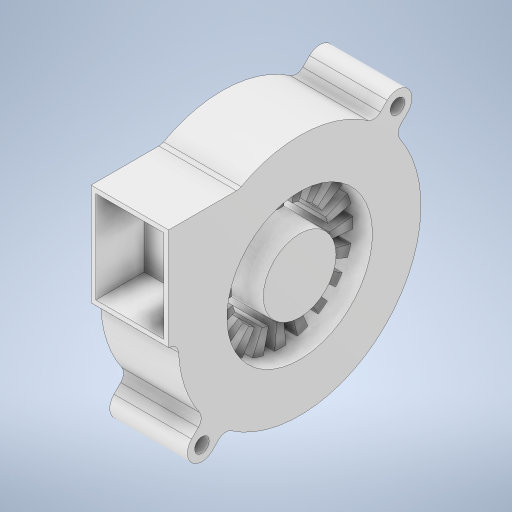
# Autodesk Inventor part: BlowerFan
Saved by Autodesk Inventor 2023 (Build 270158000, 158)
## iProperties
Created: 2023-01-18
Part Number: BlowerFan
Material: PC/ABS Plastic
Document SubType Name: Modeling
Designer: Administrator
Density: 0.357273 g/cm^3
Appearance: Smooth - White
Author: Administrator
Autodesk Inventor part; units mm, degrees
ref_plane "YZ Plane" through (0, 0, 0) normal (1, 0, 0) x (0, 1, 0)
ref_plane "XZ Plane" through (0, 0, 0) normal (0, 1, 0) x (-1, 0, 0)
ref_plane "XY Plane" through (0, 0, 0) normal (0, 0, 1) x (1, 0, 0)
sketch "Sketch1" plane through (0, 0, 0) normal (0, 0, 1) x (1, 0, 0)
  line L0 (0, 0) -> (40.3051, 0) construction
  line L1 (40.3051, 0) -> (40.3051, 40.3051) construction
  line L2 (40.3051, 40.3051) -> (0, 40.3051) construction
  line L3 (0, 40.3051) -> (0, 0) construction
  circle A0 centre (0, 0) radius 1.5
  circle A1 centre (40.3051, 40.3051) radius 1.5
  circle A2 centre (20.1525, 20.1525) radius 25
  circle A3 centre (0, 0) radius 3
  circle A4 centre (40.3051, 40.3051) radius 3
  line L4 (2.1213, -2.1213) -> (42.4264, 38.1838)
  line L5 (42.4264, 38.1838) -> (38.1838, 42.4264)
  line L6 (38.1838, 42.4264) -> (-2.1213, 2.1213)
  line L7 (-2.1213, 2.1213) -> (2.1213, -2.1213)
  line L8 (2.1213, -2.1213) -> (38.1838, 42.4264) construction
  line L9 (42.4264, 38.1838) -> (-2.1213, 2.1213) construction
  line L10 (32.6492, 41.8051) -> (-4.8475, 41.8051) construction
  line L11 (-4.8475, 41.8051) -> (-4.8475, 20.1525) construction
  line L12 (-6.8475, 41.8051) -> (7.6558, 41.8051)
  line L13 (-6.8475, 20.8051) -> (-6.8475, 41.8051)
  line L14 (-4.8389, 20.8051) -> (-6.8475, 20.8051)
  point P0 (1.1525, 41.8051)
  point P1 (35.5812, 39.8238)
  point P2 (0.4813, 4.7239)
  point P3 (4.7239, 0.4813)
  point P4 (39.8238, 35.5812)
  dimension "d0" = 40.3051
  dimension "d1" = 40.3051
  dimension "d2" = 3
  dimension "d3" = 3
  dimension "d4" = 50
  dimension "d5" = 6
  dimension "d6" = 6
  dimension "d7" = 6
  dimension "d10" = 2
  dimension "d11" = 0
  constraints: 30 end point, 5 centre point, 5 parallel, 4 coincident, 4 point on circle, 3 horizontal, 2 midpoint, 2 perpendicular, 1 tangent
  measures "d0" distance of L2.end L1.end
  measures "d1" distance of L0.end L1.end
  measures "d2" diameter of A0
  measures "d3" diameter of A1
  measures "d4" diameter of A2
  measures "d5" diameter of A3
  measures "d6" diameter of A4
  measures "d7" distance of L5.end L4.end
  measures "d10" distance between parallel lines of L11 L13
  measures "d11" distance from line of L10 point (1.153, 41.805)
extrude "Extrusion1" add sketch "Sketch1" along normal blind 16 contours A0 L7 A3 | A0 L7 A3 | L6 A2 L4 A3 | L6 A2 L4 | A2 L6 | L4 A2 | L14 L13 L12 A2 | L6 A4 L4 A2 | L5 A1 A4 | A4 L5 A1
fillet "Fillet1" radius 2 6 edges at (-4.8389, 20.8051, 8) (0.4813, 4.7239, 8) (4.7239, 0.4813, 8) (7.6558, 41.8051, 8) (35.5812, 39.8238, 8) (39.8238, 35.5812, 8)
sketch "Sketch4" plane through (-6.8475, 20.8051, 0) normal (-1, 0, 0) x (0, 0, 1)
  line L0 (0, 21) -> (0, 0) construction
  line L1 (0, 21) -> (16, 21) construction
  line L2 (0, 0) -> (16, 21) construction
  line L3 (1, 1) -> (15, 1)
  line L4 (15, 1) -> (15, 20)
  line L5 (15, 20) -> (1, 20)
  line L6 (1, 20) -> (1, 1)
  line L7 (1, 1) -> (15, 20) construction
  line L8 (15, 1) -> (1, 20) construction
  point P0 (0, -20.8051)
  point P1 (8, 10.5)
  dimension "d31" = 14
  dimension "d32" = 19
  constraints: 14 end point, 3 midpoint, 2 parallel, 1 horizontal, 1 perpendicular
  measures "d31" distance of L5.end L4.end
  measures "d32" distance of L4.end L3.end
extrude "Extrusion4" cut sketch "Sketch4" against normal blind 10
sketch "Sketch2" plane through (0, 0, 16) normal (0, 0, 1) x (1, 0, 0)
  arc A0 (6.0543, -0.493) -> (40.7981, 34.2508) centre (20.1525, 20.1525) ccw projected
  circle A1 centre (20.1525, 20.1525) radius 15
  circle A2 centre (20.1525, 20.1525) radius 7.5
  point P0 (0, 0)
  dimension "d15" = 30
  dimension "d16" = 15
  constraints: 2 centre point, 2 coincident
  measures "d15" diameter of A1
  measures "d16" diameter of A2
extrude "Extrusion2" cut sketch "Sketch2" against normal blind 14
sketch "Sketch3" plane through (20.1525, 20.1525, 2) normal (0, 0, 1) x (1, 0, 0)
  circle A0 centre (0, -0.0295) radius 15 construction
  circle A1 centre (0, -0.0295) radius 7.5 construction
  line L0 (0, 7.4705) -> (-0.5, 7.4705)
  line L1 (0, 7.4705) -> (0.5, 7.4705) construction
  line L2 (-0.5, 7.4705) -> (-1.1523, 14.9262)
  line L3 (0, 7.4705) -> (0.5, 7.4705)
  line L4 (0.5, 7.4705) -> (1.1523, 14.9262)
  line L5 (0.7278, 10.0744) -> (-0.7278, 10.0744)
  arc A2 (1.1523, 14.9262) -> (-1.1523, 14.9262) centre (0, -0.0295) ccw
  point P0 (-20.1525, -20.1525)
  dimension "d20" = 15
  dimension "d19" = 30
  dimension "d21" = 0.5
  dimension "d22" = 180
  dimension "d23" = 95
  dimension "d24" = 0.5
  dimension "d25" = 95
  constraints: 12 end point, 5 horizontal, 4 point on circle, 2 centre point, 2 point on line, 1 coincident, 1 collinear, 1 concentric, 1 vertical alignment, 2 other
  measures "d19" diameter of A0
  measures "d21" distance of L0.start L0.end
  measures "d22" angle of L0 L1
  measures "d23" angle of L0 L2
  measures "d24" distance of L0.start L1.end
  measures "d25" angle of L4 L3
extrude "Extrusion3" add sketch "Sketch3" along normal blind 10 contours L2 A2 L4 L5
pattern_circular "Circular Pattern1" count 20 over 360 about axis through (20.1525, 20.1525, 16) along (0, 0, -1) of "Extrusion3"
equation "\"d1\" = d0"
body "Solid1"
